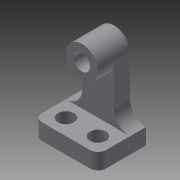
# Autodesk Inventor part: 7.1 Q5
Saved by Autodesk Inventor 2015 (Build 190159000, 159)
## iProperties
Created: 2018-02-08
Part Number: 7.1 Q5
Material: Generic
Document SubType Name: Modeling
Designer: Administrator
Density: 1 g/cm^3
Appearance: Default
Author: Administrator
Autodesk Inventor part; units mm, degrees
ref_plane "YZ Plane" through (0, 0, 0) normal (1, 0, 0) x (0, 1, 0)
ref_plane "XZ Plane" through (0, 0, 0) normal (0, 1, 0) x (-1, 0, 0)
ref_plane "XY Plane" through (0, 0, 0) normal (0, 0, 1) x (1, 0, 0)
sketch "Sketch1" plane through (0, 0, 0) normal (0, 0, 1) x (1, 0, 0)
  line L0 (0, 12.7) -> (0, 0)
  line L1 (0, 0) -> (50.8, 0)
  line L2 (50.8, 0) -> (50.8, 12.7)
  line L3 (0, 12.7) -> (12.7, 12.7)
  line L4 (50.8, 12.7) -> (38.1, 12.7)
  line L5 (12.7, 12.7) -> (12.7, 57.15)
  line L6 (38.1, 12.7) -> (38.1, 57.15)
  arc A0 (38.1, 57.15) -> (12.7, 57.15) centre (25.4, 57.15) ccw
  dimension "d0" = 50.8
  dimension "d1" = 12.7
  dimension "d2" = 12.7
  dimension "d3" = 12.7
  dimension "d5" = 12.7
  dimension "d6" = 44.45
  constraints: 14 end point, 3 vertical, 2 horizontal, 2 point on circle, 1 centre point, 1 perpendicular
  measures "d0" distance of L0.end L1.end
  measures "d1" distance of L0.start L0.end
  measures "d2" distance of L0.start L3.end
  measures "d3" distance of L2.end L4.end
  measures "d5" radius of A0
  measures "d6" distance of L3.end L5.end
extrude "Extrusion1" add sketch "Sketch1" along normal blind 38.1
fillet "Fillet1" radius 6.35 2 edges at (50.8, 6.35, 38.1) (0, 6.35, 38.1)
sketch "Sketch2" plane through (0, 0, 38.1) normal (0, 0, 1) x (1, 0, 0)
  arc A0 (12.7, 57.15) -> (38.1, 57.15) centre (25.4, 57.15) ccw
  line L0 (12.7, 57.15) -> (12.7, 12.7)
  line L1 (12.7, 57.15) -> (12.7, 12.7) projected
  line L2 (12.7, 12.7) -> (38.1, 12.7)
  line L3 (38.1, 12.7) -> (38.1, 57.15)
  point P0 (0, 0)
  constraints: 6 end point, 2 perpendicular, 2 point on circle, 2 tangent, 1 centre point, 1 collinear
sketch "Sketch2 outline for Extrusion2" plane through (0, 0, 38.1) normal (0, 0, 1) x (1, 0, 0)
  arc A0 (38.1, 57.15) -> (12.7, 57.15) centre (25.4, 57.15) cw
  line L0 (38.1, 12.7) -> (38.1, 57.15)
  line L1 (12.7, 12.7) -> (38.1, 12.7)
  line L2 (12.7, 57.15) -> (12.7, 12.7)
extrude "Extrusion2" cut sketch "Sketch2 outline for Extrusion2" against normal blind 25.4
sketch "Sketch3" plane through (25.4, 57.15, 38.1) normal (0, 0, 1) x (1, 0, 0)
  circle A0 centre (0, 0) radius 12.7
  point P0 (-25.4, -57.15)
  constraints: 1 centre point
extrude "Extrusion3" cut sketch "Sketch3" against normal blind 12.7
hole "Hole1" at (25.4, 57.15, 38.1) direction (0, 0, -1) diameter 12.7 end through all
sketch "Sketch4" plane through (38.1, 12.7, 0) normal (0, 1, 0) x (1, 0, 0)
  line L0 (6.35, -38.1) -> (-31.75, -38.1) projected
  line L1 (-38.1, 0) -> (-38.1, -31.75) projected
  line L2 (12.7, 0) -> (12.7, -31.75) projected
  point P0 (-25.4, -25.4)
  point P1 (0, -25.4)
  dimension "d21" = 12.7
  dimension "d22" = 12.7
  dimension "d23" = 12.7
  dimension "d24" = 12.7
  measures "d21" distance from line of L0 point (-25.4, -25.4)
  measures "d22" distance from line of point (-25.4, -25.4) L1
  measures "d23" distance from line of L2 point (0, -25.4)
  measures "d24" distance from line of L0 point (0, -25.4)
hole "Hole2" at (12.7, 12.7, 25.4) at (38.1, 12.7, 25.4) direction (0, -1, 0) diameter 12.7 end through all
fillet "Fillet2" radius 12.7 2 edges at (38.1, 12.7, 6.35) (12.7, 12.7, 6.35)
body "Solid1"
